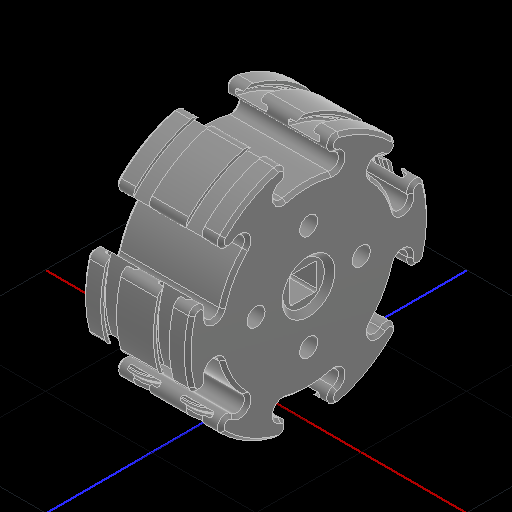
# Autodesk Inventor part: internal
Saved by Autodesk Inventor 2025.2 (Build 292293000, 293)
## iProperties
Created: 2025-11-17
Part Number: internal
Material: white pla
Document SubType Name: Modeling
Designer: cloudy
Density: 1 g/cm^3
Appearance: Smooth - Dark Gray
Author: cloudy
Autodesk Inventor part; units mm, degrees
ref_plane "YZ Plane" through (0, 0, 0) normal (1, 0, 0) x (0, 1, 0)
ref_plane "XZ Plane" through (0, 0, 0) normal (0, 1, 0) x (-1, 0, 0)
ref_plane "XY Plane" through (0, 0, 0) normal (0, 0, 1) x (1, 0, 0)
sketch "Sketch2" plane through (0, 0, 0) normal (0, 0, 1) x (1, 0, 0)
  line L0 (-12.7, 0) -> (12.7, 0)
  line L1 (-12.7, 0) -> (-12.7, 29.21)
  line L2 (-12.7, 29.21) -> (12.7, 29.21)
  line L3 (12.7, 29.21) -> (12.7, 0)
  line L4 (-10.16, 26.67) -> (-3.8407, 26.67)
  line L5 (2.54, 26.67) -> (10.16, 26.67)
  line L6 (-10.16, 26.67) -> (-10.16, 27.94)
  line L7 (-10.16, 27.94) -> (-8.255, 27.94)
  line L8 (-8.255, 27.94) -> (-8.255, 29.21)
  line L9 (-4.445, 29.21) -> (-4.445, 27.94)
  line L10 (-4.445, 27.94) -> (-2.54, 27.94)
  line L11 (-2.54, 27.94) -> (-2.54, 26.67)
  line L12 (-2.54, 26.67) -> (-3.8407, 26.67)
  line L13 (2.54, 26.67) -> (2.54, 27.94)
  line L14 (2.54, 27.94) -> (4.445, 27.94)
  line L15 (4.445, 27.94) -> (4.445, 29.21)
  line L16 (8.255, 29.21) -> (8.255, 27.94)
  line L17 (8.255, 27.94) -> (10.16, 27.94)
  line L18 (10.16, 27.94) -> (10.16, 26.67)
  line L19 (-17.78, 0) -> (17.78, 0) projected
  point P0 (0, 0)
  point P1 (-10.16, 27.305)
  dimension "d6" = 25.4
  dimension "d7" = 29.21
  dimension "d8" = 7.62
  dimension "d9" = 2.54
  dimension "d10" = 1.27
  dimension "d11" = 3.81
  dimension "d12" = 1.905
  dimension "d13" = 2.54
  dimension "d14" = 2.54
  dimension "d15" = 7.62
  dimension "d16" = 4.445
  dimension "d17" = 3.81
  constraints: 38 end point, 10 vertical, 8 horizontal, 6 point on line, 3 collinear, 2 midpoint, 1 parallel
  measures "d6" distance of L0.start L0.end
  measures "d7" distance of L0.start L1.end
  measures "d8" distance between parallel lines of L6 L11
  measures "d9" distance between parallel lines of L2 L4
  measures "d10" distance between parallel lines of L2 L7
  measures "d11" distance between parallel lines of L8 L9
  measures "d12" distance from line of point (-10.16, 27.305) L8
  measures "d13" distance between parallel lines of L1 L6
  measures "d14" distance between parallel lines of L3 L18
  measures "d15" distance of L5.start L5.end
  measures "d16" distance between parallel lines of L3 L16
  measures "d17" distance between parallel lines of L15 L16
revolve "Revolution1" add sketch "Sketch2" angle 360 about axis through (-10, 0, 0) along (1, 0, 0) contours L1 L2 L8 L7 L6 L4 L12 L11 L10 L9 L15 L14 L13 L5 L18 L17 L16 L3 L0
fillet "Fillet1" radius 0.5 12 edges at (4.445, -27.94, 0) (2.54, -27.94, 0) (2.54, -26.67, 0) (-4.445, -27.94, 0) (-2.54, -27.94, 0) (-2.54, -26.67, 0) (-8.255, -27.94, 0) (-10.16, -27.94, 0) (-10.16, -26.67, 0) (8.255, -27.94, 0) (10.16, -27.94, 0) (10.16, -26.67, 0)
sketch "Sketch3" plane through (-12.7, 0, 0) normal (-1, 0, 0) x (0, 0, 1)
  circle A0 centre (0, 0) radius 29.21 projected
  arc A1 (26.3746, -7.0671) -> (26.3746, 7.0671) centre (0, 0) ccw construction
  arc A2 (28.2147, -7.5601) -> (28.2147, 7.5601) centre (0, 0) ccw
  arc A3 (24.5345, -6.574) -> (24.5345, 6.574) centre (0, 0) ccw
  arc A4 (24.5345, -6.574) -> (28.2147, -7.5601) centre (26.3746, -7.0671) ccw
  arc A5 (28.2147, 7.5601) -> (24.5345, 6.574) centre (26.3746, 7.0671) ccw
  line L0 (0, 0) -> (26.3746, 7.0671) construction
  line L1 (0, 0) -> (27.305, 0) construction
  line L2 (0, 0) -> (26.3746, -7.0671) construction
  arc A6 (7.5601, 28.2147) -> (6.574, 24.5345) centre (7.0671, 26.3746) ccw
  arc A7 (17.9605, 17.9605) -> (6.574, 24.5345) centre (0, 0) ccw
  arc A8 (17.9605, 17.9605) -> (20.6546, 20.6546) centre (19.3076, 19.3076) ccw
  arc A9 (20.6546, 20.6546) -> (7.5601, 28.2147) centre (0, 0) ccw
  arc A10 (-20.6546, 20.6546) -> (-17.9605, 17.9605) centre (-19.3076, 19.3076) ccw
  arc A11 (-6.574, 24.5345) -> (-17.9605, 17.9605) centre (0, 0) ccw
  arc A12 (-6.574, 24.5345) -> (-7.5601, 28.2147) centre (-7.0671, 26.3746) ccw
  arc A13 (-7.5601, 28.2147) -> (-20.6546, 20.6546) centre (0, 0) ccw
  arc A14 (-28.2147, -7.5601) -> (-24.5345, -6.574) centre (-26.3746, -7.0671) ccw
  arc A15 (-24.5345, 6.574) -> (-24.5345, -6.574) centre (0, 0) ccw
  arc A16 (-24.5345, 6.574) -> (-28.2147, 7.5601) centre (-26.3746, 7.0671) ccw
  arc A17 (-28.2147, 7.5601) -> (-28.2147, -7.5601) centre (0, 0) ccw
  arc A18 (-7.5601, -28.2147) -> (-6.574, -24.5345) centre (-7.0671, -26.3746) ccw
  arc A19 (-17.9605, -17.9605) -> (-6.574, -24.5345) centre (0, 0) ccw
  arc A20 (-17.9605, -17.9605) -> (-20.6546, -20.6546) centre (-19.3076, -19.3076) ccw
  arc A21 (-20.6546, -20.6546) -> (-7.5601, -28.2147) centre (0, 0) ccw
  arc A22 (20.6546, -20.6546) -> (17.9605, -17.9605) centre (19.3076, -19.3076) ccw
  arc A23 (6.574, -24.5345) -> (17.9605, -17.9605) centre (0, 0) ccw
  arc A24 (6.574, -24.5345) -> (7.5601, -28.2147) centre (7.0671, -26.3746) ccw
  arc A25 (7.5601, -28.2147) -> (20.6546, -20.6546) centre (0, 0) ccw
  arc A26 (16.6135, -16.6135) -> (22.6944, -6.081) centre (0, 0) ccw construction
  arc A27 (17.9605, -17.9605) -> (24.5345, -6.574) centre (0, 0) ccw
  arc A28 (15.2664, -15.2664) -> (20.8543, -5.5879) centre (0, 0) ccw
  arc A29 (15.2664, -15.2664) -> (17.9605, -17.9605) centre (16.6135, -16.6135) ccw
  arc A30 (24.5345, -6.574) -> (20.8543, -5.5879) centre (22.6944, -6.081) ccw
  line L3 (22.6944, -6.081) -> (0, 0) construction
  line L4 (0, 0) -> (16.6135, -16.6135) construction
  arc A31 (17.9605, 17.9605) -> (15.2664, 15.2664) centre (16.6135, 16.6135) ccw
  arc A32 (24.5345, 6.574) -> (17.9605, 17.9605) centre (0, 0) ccw
  arc A33 (20.8543, 5.5879) -> (15.2664, 15.2664) centre (0, 0) ccw
  arc A34 (20.8543, 5.5879) -> (24.5345, 6.574) centre (22.6944, 6.081) ccw
  arc A35 (-6.574, 24.5345) -> (-5.5879, 20.8543) centre (-6.081, 22.6944) ccw
  arc A36 (6.574, 24.5345) -> (-6.574, 24.5345) centre (0, 0) ccw
  arc A37 (5.5879, 20.8543) -> (-5.5879, 20.8543) centre (0, 0) ccw
  arc A38 (5.5879, 20.8543) -> (6.574, 24.5345) centre (6.081, 22.6944) ccw
  arc A39 (-24.5345, 6.574) -> (-20.8543, 5.5879) centre (-22.6944, 6.081) ccw
  arc A40 (-17.9605, 17.9605) -> (-24.5345, 6.574) centre (0, 0) ccw
  arc A41 (-15.2664, 15.2664) -> (-20.8543, 5.5879) centre (0, 0) ccw
  arc A42 (-15.2664, 15.2664) -> (-17.9605, 17.9605) centre (-16.6135, 16.6135) ccw
  arc A43 (-17.9605, -17.9605) -> (-15.2664, -15.2664) centre (-16.6135, -16.6135) ccw
  arc A44 (-24.5345, -6.574) -> (-17.9605, -17.9605) centre (0, 0) ccw
  arc A45 (-20.8543, -5.5879) -> (-15.2664, -15.2664) centre (0, 0) ccw
  arc A46 (-20.8543, -5.5879) -> (-24.5345, -6.574) centre (-22.6944, -6.081) ccw
  arc A47 (6.574, -24.5345) -> (5.5879, -20.8543) centre (6.081, -22.6944) ccw
  arc A48 (-6.574, -24.5345) -> (6.574, -24.5345) centre (0, 0) ccw
  arc A49 (-5.5879, -20.8543) -> (5.5879, -20.8543) centre (0, 0) ccw
  arc A50 (-5.5879, -20.8543) -> (-6.574, -24.5345) centre (-6.081, -22.6944) ccw
  point P0 (20.6546, -20.6546)
  point P1 (28.2147, -7.5601)
  point P2 (23.7634, -4.1901)
  point P3 (28.2147, 7.5601)
  point P4 (20.6546, 20.6546)
  point P5 (17.9605, 17.9605)
  point P6 (6.574, 24.5345)
  point P7 (7.5601, 28.2147)
  point P8 (-7.5601, 28.2147)
  point P9 (-6.574, 24.5345)
  point P10 (-17.9605, 17.9605)
  point P11 (-20.6546, 20.6546)
  point P12 (-28.2147, 7.5601)
  point P13 (-24.5345, 6.574)
  point P14 (-24.5345, -6.574)
  point P15 (-28.2147, -7.5601)
  point P16 (-20.6546, -20.6546)
  point P17 (-17.9605, -17.9605)
  point P18 (-6.574, -24.5345)
  point P19 (7.5601, -28.2147)
  point P20 (6.574, -24.5345)
  point P21 (17.9605, -17.9605)
  point P22 (23.4385, -5.7354)
  point P23 (24.5345, -6.574)
  point P24 (17.9605, -17.9605)
  point P25 (24.5345, -6.574)
  point P26 (17.9605, -17.9605)
  point P27 (7.5601, -28.2147)
  point P28 (24.5345, -6.574)
  point P29 (24.5345, -6.574)
  point P30 (6.574, -24.5345)
  point P31 (-6.574, -24.5345)
  point P32 (-17.9605, -17.9605)
  point P33 (-24.5345, 6.574)
  point P34 (-17.9605, 17.9605)
  point P35 (6.574, 24.5345)
  point P36 (24.5345, 6.574)
  dimension "d20" = 27.305
  dimension "d21" = 15
  dimension "d22" = 30
  dimension "d23" = 3.81
  dimension "d26" = 360
  dimension "d28" = 1.905
  dimension "d29" = 30
  dimension "d33" = 360
  constraints: 100 point on circle, 50 centre point, 10 end point, 8 tangent, 2 coincident, 2 concentric, 1 collinear, 1 equal length, 1 horizontal, 134 other
  measures "d20" radius of A1
  measures "d21" angle of L1 L0
  measures "d22" angle of L2 L0
  measures "d23" diameter of A4
  measures "d28" radius of A29
  measures "d29" angle of L4 L3
extrude "Extrusion2" cut sketch "Sketch3" against normal through all contours A5 A32 A8 A0 | A0 A22 A27 A4 | A34 A33 A31 A32 | A27 A29 A28 A30 | A6 A36 A12 A0 | A0 A18 A48 A24 | A38 A37 A35 A36 | A48 A50 A49 A47 | A10 A40 A16 A0 | A0 A14 A44 A20 | A42 A41 A39 A40 | A44 A46 A45 A43
sketch "Sketch4" plane through (-12.7, 0, 0) normal (-1, 0, 0) x (0, 0, 1)
  line L0 (-3.2258, 3.2258) -> (3.2258, 3.2258)
  line L1 (3.2258, 3.2258) -> (3.2258, -3.2258)
  line L2 (3.2258, -3.2258) -> (-3.2258, -3.2258)
  line L3 (-3.2258, -3.2258) -> (-3.2258, 3.2258)
  line L4 (-3.2258, 3.2258) -> (3.2258, -3.2258) construction
  line L5 (3.2258, 3.2258) -> (-3.2258, -3.2258) construction
  point P0 (0, 0)
  dimension "d37" = 6.4516
  dimension "d38" = 6.4516
  constraints: 12 end point, 2 midpoint, 2 parallel, 1 horizontal, 1 perpendicular
  measures "d37" distance of L1.end L2.end
  measures "d38" distance of L0.end L1.end
extrude "Extrusion3" cut sketch "Sketch4" against normal through all
fillet "Fillet2" radius 0.508 4 edges at (0, -3.2258, 3.2258) (0, -3.2258, -3.2258) (0, 3.2258, -3.2258) (0, 3.2258, 3.2258)
sketch "Sketch5" plane through (-12.7, 0, 0) normal (-1, 0, 0) x (0, 0, 1)
  circle A0 centre (0, 0) radius 5.08
  dimension "d42" = 10.16
  constraints: 1 centre point, 1 coincident
  measures "d42" diameter of A0
extrude "Extrusion4" cut sketch "Sketch5" against normal blind 1.27
chamfer "Chamfer1" distance 1.27 angle 45 1 edges at (-12.7, 0, -5.08)
sketch "Sketch6" plane through (12.7, 0, 0) normal (1, 0, 0) x (0, 0, -1)
  circle A0 centre (0, 0) radius 5.08
  dimension "d48" = 10.16
  constraints: 1 centre point, 1 coincident
  measures "d48" diameter of A0
extrude "Extrusion5" cut sketch "Sketch6" against normal blind 1.27
chamfer "Chamfer2" distance 1.27 angle 45 1 edges at (12.7, 0, 5.08)
sketch "Sketch7" plane through (12.7, 0, 0) normal (1, 0, 0) x (0, 0, -1)
  circle A0 centre (12.7, 0) radius 2.1844
  line L0 (12.7, 0) -> (0, 0) construction
  dimension "d54" = 4.3688
  dimension "d55" = 12.7
  constraints: 2 end point, 1 centre point, 1 horizontal
  measures "d54" diameter of A0
  measures "d55" distance of L0.start L0.end
extrude "Extrusion6" cut sketch "Sketch7" against normal through all
sketch "Sketch8" plane through (-12.7, 0, 0) normal (-1, 0, 0) x (0, 0, 1)
  circle A0 centre (-12.7, 0) radius 2.1844 projected
  line L0 (-8.4836, -2.4343) -> (-12.7, -4.8687)
  line L1 (-12.7, -4.8687) -> (-16.9164, -2.4343)
  line L2 (-16.9164, -2.4343) -> (-16.9164, 2.4343)
  line L3 (-16.9164, 2.4343) -> (-12.7, 4.8687)
  line L4 (-12.7, 4.8687) -> (-8.4836, 2.4343)
  line L5 (-8.4836, 2.4343) -> (-8.4836, -2.4343)
  circle A1 centre (-12.7, 4.8687) radius 0.5
  circle A2 centre (-8.4836, 2.4343) radius 0.5
  circle A3 centre (-8.4836, -2.4343) radius 0.5
  circle A4 centre (-12.7, -4.8687) radius 0.5
  circle A5 centre (-16.9164, -2.4343) radius 0.5
  circle A6 centre (-16.9164, 2.4343) radius 0.5
  point P0 (0, 0)
  point P1 (-16.9164, -1.9343)
  point P2 (-16.4834, -2.6843)
  point P3 (-13.133, -4.6187)
  point P4 (-12.267, -4.6187)
  point P5 (-8.9166, -2.6843)
  point P6 (-8.4836, -1.9343)
  point P7 (-8.4836, 1.9343)
  point P8 (-8.9166, 2.6843)
  point P9 (-12.267, 4.6187)
  point P10 (-13.133, 4.6187)
  point P11 (-16.4834, 2.6843)
  point P12 (-16.9164, 1.9343)
  dimension "d58" = 8.4328
  dimension "d59" = 1
  constraints: 12 end point, 7 coincident, 6 centre point, 5 equal radius, 1 vertical, 13 other
  measures "d58" distance between parallel lines of L2 L5
  measures "d59" diameter of A1
extrude "Extrusion7" cut sketch "Sketch8" against normal blind 4.2333 contours A0 | L5 A3 L0 | L0 A3 L5 | L0 A4 L1 A5 L2 A6 L3 A1 L4 A2 L5 A3 | A4 L1 L0 | L0 L1 A4 | A2 L4 L5 | L5 L4 A2 | A5 L2 L1 | L1 L2 A5 | A1 L3 L4 | L4 L3 A1 | A6 L3 L2 | L2 L3 A6
fillet "Fillet3" radius 3.175 12 edges at (-10.5833, 4.6187, -12.267) (-10.5833, 4.6187, -13.133) (-10.5833, 2.6843, -8.9166) (-10.5833, 1.9343, -8.4836) (-10.5833, 2.6843, -16.4834) (-10.5833, 1.9343, -16.9164) (-10.5833, -1.9343, -16.9164) (-10.5833, -2.6843, -16.4834) (-10.5833, -4.6187, -13.133) (-10.5833, -4.6187, -12.267) (-10.5833, -2.6843, -8.9166) (-10.5833, -1.9343, -8.4836)
pattern_circular "Circular Pattern1" count 4 over 360 about axis through (-12.7, 0, 0) along (1, 0, 0) of "Extrusion7", "Extrusion6", "Fillet3"
chamfer "Chamfer3" distance 0.7937 angle 45 72 edges at (-12.7, 22.2014, -7.921) (-12.7, 26.8677, -5.227) (-12.7, 25.2966, -14.605) (-12.7, 17.9605, -20.6546) (-12.7, 17.9605, -15.2664) (-12.7, 10.795, -18.6975) (-12.7, 4.2409, -23.1875) (-12.7, 8.9071, -25.8816) (-12.7, 0, -29.21) (-12.7, -8.9071, -25.8816) (-12.7, -4.2409, -23.1875) (-12.7, -10.795, -18.6975) (-12.7, -17.9605, -15.2664) (-12.7, -17.9605, -20.6546) (-12.7, -25.2966, -14.605) (-12.7, -26.8677, -5.227) (-12.7, -22.2014, -7.921) (-12.7, -21.59, 0) (-12.7, -22.2014, 7.921) (-12.7, -26.8677, 5.227) (-12.7, -25.2966, 14.605) (-12.7, -17.9605, 20.6546) (-12.7, -17.9605, 15.2664) (-12.7, -10.795, 18.6975) (-12.7, -4.2409, 23.1875) (-12.7, -8.9071, 25.8816) (-12.7, 0, 29.21) (-12.7, 8.9071, 25.8816) (-12.7, 4.2409, 23.1875) (-12.7, 10.795, 18.6975) (-12.7, 17.9605, 15.2664) (-12.7, 17.9605, 20.6546) (-12.7, 25.2966, 14.605) (-12.7, 26.8677, 5.227) (-12.7, 22.2014, 7.921) (-12.7, 21.59, 0) (12.7, 17.9605, 15.2664) (12.7, 10.795, 18.6975) (12.7, 4.2409, 23.1875) (12.7, 8.9071, 25.8816) (12.7, 0, 29.21) (12.7, -8.9071, 25.8816) (12.7, -4.2409, 23.1875) (12.7, -10.795, 18.6975) (12.7, -17.9605, 15.2664) (12.7, -17.9605, 20.6546) (12.7, -25.2966, 14.605) (12.7, -26.8677, 5.227) (12.7, -22.2014, 7.921) (12.7, -21.59, 0) (12.7, -22.2014, -7.921) (12.7, -26.8677, -5.227) (12.7, -25.2966, -14.605) (12.7, -17.9605, -20.6546) (12.7, -17.9605, -15.2664) (12.7, -10.795, -18.6975) (12.7, -4.2409, -23.1875) (12.7, -8.9071, -25.8816) (12.7, 0, -29.21) (12.7, 8.9071, -25.8816) (12.7, 4.2409, -23.1875) (12.7, 10.795, -18.6975) (12.7, 17.9605, -15.2664) (12.7, 17.9605, -20.6546) (12.7, 25.2966, -14.605) (12.7, 26.8677, -5.227) (12.7, 22.2014, -7.921) (12.7, 21.59, 0) (12.7, 22.2014, 7.921) (12.7, 26.8677, 5.227) (12.7, 25.2966, 14.605) (12.7, 17.9605, 20.6546)
body "Solid2"
